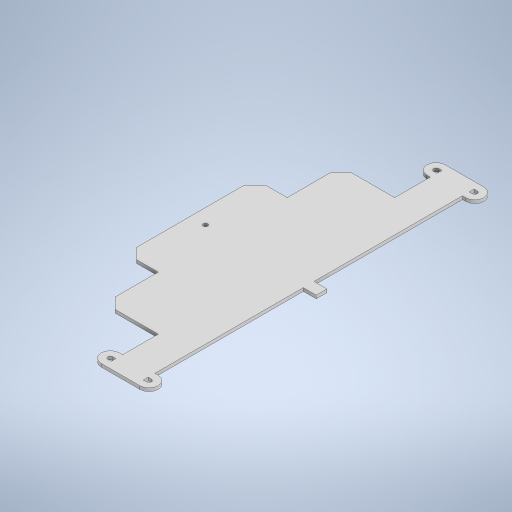
# Autodesk Inventor part: linefollower_chassy_model_3
Saved by Autodesk Inventor 2024 (Build 280153000, 153)
## iProperties
Created: 2024-02-27
Part Number: linefollower_chassy_model_3
Material: Generic
Document SubType Name: Modeling
Designer: kamil
Density: 1 g/cm^3
Appearance: Default
Author: kamil
Autodesk Inventor part; units mm, degrees
ref_plane "YZ Plane" through (0, 0, 0) normal (1, 0, 0) x (0, 1, 0)
ref_plane "XZ Plane" through (0, 0, 0) normal (0, 1, 0) x (-1, 0, 0)
ref_plane "XY Plane" through (0, 0, 0) normal (0, 0, 1) x (1, 0, 0)
sketch "Sketch1" plane through (0, 0, 0) normal (0, 1, 0) x (-1, 0, 0)
  line L0 (7.5, 80) -> (-7.5, 80)
  line L1 (-7.5, 80) -> (-7.5, -80)
  line L2 (-7.5, -80) -> (7.5, -80)
  line L3 (7.5, -80) -> (7.5, 80)
  line L4 (7.5, 80) -> (-7.5, -80) construction
  line L5 (7.5, -80) -> (-7.5, 80) construction
  line L6 (7.5, 75.75) -> (9, 75.75)
  line L7 (7.5, 80) -> (9, 80)
  line L8 (7.5, 71.5) -> (9, 71.5)
  arc A0 (9, 71.5) -> (9, 80) centre (9, 75.75) ccw
  line L9 (7.5, 74.6) -> (9, 74.6)
  line L10 (7.5, 76.9) -> (9, 76.9)
  arc A1 (9, 74.6) -> (9, 76.9) centre (9, 75.75) ccw
  line L11 (0, 80) -> (0, -80) construction
  line L12 (7.5, 0) -> (-7.5, 0) construction
  line L13 (-7.5, 75.75) -> (-9, 75.75)
  line L14 (-7.5, 80) -> (-9, 80)
  line L15 (-7.5, 71.5) -> (-9, 71.5)
  arc A2 (-9, 80) -> (-9, 71.5) centre (-9, 75.75) ccw
  line L16 (-7.5, 74.6) -> (-9, 74.6)
  line L17 (-7.5, 76.9) -> (-9, 76.9)
  arc A3 (-9, 76.9) -> (-9, 74.6) centre (-9, 75.75) ccw
  line L18 (7.5, -75.75) -> (9, -75.75)
  line L19 (7.5, -80) -> (9, -80)
  line L20 (7.5, -71.5) -> (9, -71.5)
  arc A4 (9, -80) -> (9, -71.5) centre (9, -75.75) ccw
  line L21 (7.5, -74.6) -> (9, -74.6)
  line L22 (7.5, -76.9) -> (9, -76.9)
  arc A5 (9, -76.9) -> (9, -74.6) centre (9, -75.75) ccw
  arc A6 (-9, -71.5) -> (-9, -80) centre (-9, -75.75) ccw
  line L23 (-7.5, -71.5) -> (-9, -71.5)
  line L24 (-7.5, -74.6) -> (-9, -74.6)
  arc A7 (-9, -74.6) -> (-9, -76.9) centre (-9, -75.75) ccw
  line L25 (-7.5, -75.75) -> (-9, -75.75)
  line L26 (-7.5, -76.9) -> (-9, -76.9)
  line L27 (-7.5, -80) -> (-9, -80)
  line L28 (7.5, 55) -> (27.5, 55)
  line L29 (32.5, 50) -> (32.5, 30)
  line L30 (32.5, 30) -> (42.5, 30)
  line L31 (47.5, 25) -> (47.5, 0)
  line L32 (64.2072, 0) -> (-38.11, 0) construction
  line L33 (7.5, -55) -> (27.5, -55)
  line L34 (32.5, -50) -> (32.5, -30)
  line L35 (32.5, -30) -> (42.5, -30)
  line L36 (47.5, -25) -> (47.5, 0)
  line L37 (27.5, 55) -> (32.5, 50)
  line L38 (42.5, 30) -> (47.5, 25)
  line L39 (47.5, -25) -> (42.5, -30)
  line L40 (32.5, -50) -> (27.5, -55)
  circle A8 centre (40.5, 0) radius 1.025
  circle A9 centre (-11.5, 0) radius 1.025
  line L41 (-7.5, 2.5) -> (-13.5, 2.5)
  line L42 (-13.5, 2.5) -> (-13.5, -2.5)
  line L43 (-13.5, -2.5) -> (-7.5, -2.5)
  line L44 (-7.5, -2.5) -> (-7.5, 2.5)
  point P0 (0, 0)
  point P1 (0, 0)
  point P2 (8.25, 71.5)
  point P3 (32.5, 55)
  point P4 (47.5, 30)
  point P5 (32.5, -55)
  point P6 (47.5, -30)
  dimension "d0" = 160
  dimension "d1" = 15
  dimension "d2" = 1.5
  dimension "d3" = 4.25
  dimension "d5" = 4.25
  dimension "d6" = 4.25
  dimension "d7" = 1.15
  dimension "d8" = 1.15
  dimension "d9" = 1.15
  dimension "d10" = 25
  dimension "d11" = 25
  dimension "d12" = 15
  dimension "d13" = 25
  dimension "d14" = 25
  dimension "d15" = 5
  dimension "d16" = 5
  dimension "d17" = 5
  dimension "d18" = 5
  dimension "d19" = 5
  dimension "d20" = 5
  dimension "d21" = 5
  dimension "d22" = 5
  dimension "d24" = 2.05
  dimension "d25" = 7
  dimension "d26" = 2.05
  dimension "d27" = 4
  dimension "d28" = 2.5
  dimension "d29" = 2.5
  dimension "d30" = 6
  constraints: 90 end point, 37 symmetric about line, 16 point on circle, 16 point on line, 10 centre point, 9 coincident, 8 horizontal, 6 midpoint, 4 parallel, 4 perpendicular, 2 vertical, 6 other
  measures "d0" distance of L2.end L0.start
  measures "d1" distance between parallel lines of L1 L3
  measures "d2" distance of L6.start L6.end
  measures "d3" distance between parallel lines of L0 L6
  measures "d5" distance from line of L6 point (8.25, 71.5)
  measures "d6" radius of A0
  measures "d7" distance between parallel lines of L9 L6
  measures "d8" distance between parallel lines of L6 L10
  measures "d9" radius of A1
  measures "d10" distance of L28.start point (32.5, 55)
  measures "d11" distance of point (32.5, 55) L29.end
  measures "d12" distance of L29.end point (47.5, 30)
  measures "d13" distance between parallel lines of L0 L28
  measures "d14" distance between parallel lines of L2 L33
  measures "d15" distance of L28.end point (32.5, 55)
  measures "d16" distance of L29.start point (32.5, 55)
  measures "d17" distance of L30.end point (47.5, 30)
  measures "d18" distance of L31.start point (47.5, 30)
  measures "d19" distance of L36.start point (47.5, -30)
  measures "d20" distance of L35.end point (47.5, -30)
  measures "d21" distance of L34.start point (32.5, -55)
  measures "d22" distance of L33.end point (32.5, -55)
  measures "d24" diameter of A8
  measures "d25" distance from line of A8.centre L36
  measures "d26" diameter of A9
  measures "d27" distance from line of L1 A9.centre
  measures "d28" distance between parallel lines of L32 L41
  measures "d29" distance between parallel lines of L32 L43
  measures "d30" distance between parallel lines of L1 L42
extrude "Extrusion1" add sketch "Sketch1" along normal blind 1.5 contours L3 L2 L1 L0 | L7 A0 L8 L3 L9 A1 L10 | L1 L17 A3 L16 L15 A2 L14 | L28 L37 L29 L30 L38 L31 L36 L39 L35 L34 L40 L33 L3 | L1 L43 L42 L41 | L20 A4 L19 L3 L22 A5 L21 | L1 L24 A7 L26 L27 A6 L23 | A9
equation "\"d16\" = d15"
equation "\"d17\" = d15"
equation "\"d18\" = d17"
equation "\"d19\" = d15"
equation "\"d20\" = d19"
equation "\"d21\" = d15"
equation "\"d22\" = d21"
body "Solid1"
